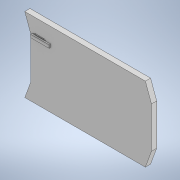
# Autodesk Inventor part: ДИ 00.00.03
Saved by Autodesk Inventor 2021.2 (Build 252289000, 289)
## iProperties
Created: 2021-10-11
Part Number: ДИ 00.00.03
Material: Типовые
Document SubType Name: Modeling
Designer: Surflay
Density: 1 g/cm^3
Appearance: По умолчанию
Author: Surflay
Autodesk Inventor part; units mm, degrees
ref_plane "YZ Plane" through (0, 0, 0) normal (1, 0, 0) x (0, 1, 0)
ref_plane "XZ Plane" through (0, 0, 0) normal (0, 1, 0) x (-1, 0, 0)
ref_plane "XY Plane" through (0, 0, 0) normal (0, 0, 1) x (1, 0, 0)
sketch "Эскиз1" plane through (0, 0, 0) normal (0, 0, 1) x (1, 0, 0)
  line L0 (0, 0) -> (170, 0)
  line L1 (170, 0) -> (170, 100)
  line L2 (170, 100) -> (0, 100)
  line L3 (0, 100) -> (0, 0) construction
  line L4 (0, 100) -> (8.1893, 77.5)
  line L5 (8.1893, 77.5) -> (8.1893, 22.5)
  line L6 (8.1893, 22.5) -> (0, 0)
  line L7 (161.8107, 100) -> (170, 77.5)
  line L8 (170, 22.5) -> (161.8107, 0)
  dimension "d0" = 170
  dimension "d1" = 100
  dimension "d2" = 20
  dimension "d3" = 55
  dimension "d4" = 20
  dimension "d6" = 55
  dimension "d7" = 20
  constraints: 18 end point, 4 point on line, 3 parallel, 1 horizontal, 1 horizontal alignment, 1 perpendicular, 1 vertical
  measures "d0" distance of L2.end L1.end
  measures "d1" distance of L1.end L0.end
  measures "d2" angle of L3 L4
  measures "d3" distance of L4.end L5.end
  measures "d4" angle of L3 L6
  measures "d6" distance of L7.end L8.start
  measures "d7" angle of L1 L7
extrude "Выдавливание1" add sketch "Эскиз1" against normal blind 7 contours L6 L5 L4 L2 L7 L1 L8 L0
sketch "Эскиз2" plane through (0, 0, 0) normal (0, 0, 1) x (1, 0, 0)
  line L0 (14.0981, 75.5) -> (25.0981, 75.5)
  line L1 (27.0981, 77.5) -> (27.0981, 77.5)
  line L2 (25.0981, 79.5) -> (14.0981, 79.5)
  line L3 (12.0981, 77.5) -> (12.0981, 77.5)
  line L4 (12.0981, 75.5) -> (27.0981, 79.5) construction
  line L5 (27.0981, 75.5) -> (12.0981, 79.5) construction
  arc A0 (14.0981, 79.5) -> (12.0981, 77.5) centre (14.0981, 77.5) ccw
  arc A1 (12.0981, 77.5) -> (14.0981, 75.5) centre (14.0981, 77.5) ccw
  arc A2 (25.0981, 75.5) -> (27.0981, 77.5) centre (25.0981, 77.5) ccw
  arc A3 (27.0981, 77.5) -> (25.0981, 79.5) centre (25.0981, 77.5) ccw
  point P0 (0, 0)
  point P1 (19.5981, 77.5)
  dimension "d10" = 15
  dimension "d11" = 4
  dimension "d12" = 2
  constraints: 12 end point, 8 point on circle, 8 point on line, 8 tangent, 4 centre point, 3 equal radius, 2 midpoint, 2 parallel, 1 horizontal, 1 perpendicular
  measures "d10" distance of L5.end L4.end
  measures "d11" distance of L4.end L5.start
  measures "d12" radius of A0
extrude "Выдавливание2" cut sketch "Эскиз2" against normal blind 2
fillet "Сопряжение1" radius 2 4 edges at (27.0981, 77.5, 0) (19.5981, 75.5, 0) (12.0981, 77.5, 0) (19.5981, 79.5, 0)
fillet "Сопряжение2" radius 2 8 edges at (19.5981, 79.5, -1.9995) (19.5981, 79.5, -2) (27.0981, 77.5, -1.9995) (27.0981, 77.5, -2) (19.5981, 75.5, -1.9995) (19.5981, 75.5, -2) (12.0981, 77.5, -1.9995) (12.0981, 77.5, -2)
sketch "Эскиз3" plane through (0, 0, 0) normal (0, 0, 1) x (1, 0, 0)
  line L0 (9.6893, 79.5) -> (34.6893, 79.5)
  line L1 (34.6893, 79.5) -> (34.6893, 75.5)
  line L2 (34.6893, 75.5) -> (9.6893, 75.5)
  line L3 (9.6893, 75.5) -> (9.6893, 79.5)
  line L4 (14.0981, 73.5) -> (25.0981, 73.5) projected
  line L5 (8.1893, 77.5) -> (8.1893, 22.5) projected
  point P0 (0, 0)
  dimension "d17" = 4
  dimension "d18" = 25
  dimension "d19" = 2
  dimension "d20" = 1.5
  constraints: 8 end point, 2 parallel, 1 horizontal, 1 perpendicular
  measures "d17" distance between parallel lines of L2 L0
  measures "d18" distance between parallel lines of L1 L3
  measures "d19" distance between parallel lines of L4 L2
  measures "d20" distance between parallel lines of L5 L3
extrude "Выдавливание3" add sketch "Эскиз3" along normal blind 2
